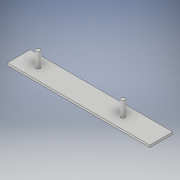
# Autodesk Inventor part: DinRail
Saved by Autodesk Inventor 2017 (Build 210142000, 142)
## iProperties
Created: 2017-02-10
Part Number: DinRail
Material: Generic
Document SubType Name: Modeling
Designer: michael
Density: 1 g/cm^3
Appearance: Default
Author: michael
Autodesk Inventor part; units mm, degrees
ref_plane "YZ Plane" through (0, 0, 0) normal (1, 0, 0) x (0, 1, 0)
ref_plane "XZ Plane" through (0, 0, 0) normal (0, 1, 0) x (-1, 0, 0)
ref_plane "XY Plane" through (0, 0, 0) normal (0, 0, 1) x (1, 0, 0)
sketch "Sketch1" plane through (0, 0, 0) normal (0, 1, 0) x (-1, 0, 0)
  line L0 (0, 0) -> (167.4876, 0)
  line L1 (167.4876, 0) -> (167.4876, -27)
  line L2 (167.4876, -27) -> (0, -27)
  line L3 (0, -27) -> (0, 0)
  dimension "d0" = 167.4876
  dimension "d1" = 27
  constraints: 8 end point, 2 parallel, 1 horizontal, 1 perpendicular
  measures "d0" distance of L1.end L2.end
  measures "d1" distance of L0.end L1.end
extrude "Extrusion1" add sketch "Sketch1" along normal blind 2.54
sketch "Sketch2" plane through (0, 2.54, 0) normal (0, 1, 0) x (1, 0, 0)
  circle A0 centre (-45, 13.5001) radius 2.5
  line L0 (-167.4876, 0) -> (0, 0) projected
  line L1 (0, 0) -> (0, 27) projected
  circle A1 centre (-145, 13.5128) radius 2.5
  dimension "d4" = 5
  dimension "d5" = 13.5001
  dimension "d6" = 45
  dimension "d7" = 5
  dimension "d8" = 13.5128
  dimension "d9" = 100
  constraints: 2 centre point
  measures "d4" diameter of A0
  measures "d5" distance from line of L0 A0.centre
  measures "d6" distance from line of A0.centre L1
  measures "d7" diameter of A1
  measures "d8" distance from line of L0 A1.centre
  measures "d9" distance of A1.centre A0.centre
extrude "Extrusion2" add sketch "Sketch2" along normal blind 17.5
body "Solid1"
